Autodesk Inventor part; units mm, degrees
(part 4 of 5)
  arc A546 (145.9727, 136.2043) -> (145.8783, 135.638) centre (153.3985, 134.6758) ccw projected
  arc A547 (146.1603, 136.9638) -> (145.9727, 136.2043) centre (155.6764, 134.2093) ccw projected
  arc A548 (146.4869, 137.9385) -> (146.1603, 136.9638) centre (158.0193, 133.5328) ccw projected
  arc A549 (147.2749, 137.9773) -> (146.4869, 137.9385) centre (148.5, 105) ccw projected
  arc A550 (147.6954, 137.0392) -> (147.2749, 137.9773) centre (136.2299, 132.4624) ccw projected
  arc A551 (147.9566, 136.3017) -> (147.6954, 137.0392) centre (138.4951, 133.3653) ccw projected
  point P0 (0, 0)
fillet "フィレット1" radius 0.5 128 edges at (167.7015, 129.018, -2.5) (168.3105, 128.5182, -2.5) (169.9632, 127.0203, -2.5) (170.5203, 126.4632, -2.5) (165.91, 130.3467, -2.5) (165.2548, 130.7845, -2.5) (163.3417, 131.9311, -2.5) (162.6468, 132.3026, -2.5) (160.6305, 133.2562, -2.5) (159.9026, 133.5577, -2.5) (157.8025, 134.3091, -2.5) (157.0485, 134.5379, -2.5) (154.8849, 135.0798, -2.5) (154.1121, 135.2335, -2.5) (151.9058, 135.5608, -2.5) (151.1217, 135.638, -2.5) (148.894, 135.7475, -2.5) (148.106, 135.7475, -2.5) (145.8783, 135.638, -2.5) (145.0942, 135.5608, -2.5) (142.8879, 135.2335, -2.5) (142.1151, 135.0798, -2.5) (139.9515, 134.5379, -2.5) (139.1975, 134.3091, -2.5) (137.0974, 133.5577, -2.5) (136.3695, 133.2562, -2.5) (134.3532, 132.3026, -2.5) (133.6583, 131.9311, -2.5) (131.7452, 130.7845, -2.5) (131.09, 130.3467, -2.5) (129.2985, 129.018, -2.5) (128.6895, 128.5182, -2.5) (127.0368, 127.0203, -2.5) (126.4797, 126.4632, -2.5) (124.9818, 124.8105, -2.5) (124.482, 124.2015, -2.5) (123.1533, 122.41, -2.5) (122.7155, 121.7548, -2.5) (121.5689, 119.8417, -2.5) (121.1974, 119.1468, -2.5) (120.2438, 117.1305, -2.5) (119.9423, 116.4026, -2.5) (118.9621, 113.5485, -2.5) (119.1909, 114.3025, -2.5) (118.4202, 111.3849, -2.5) (118.2665, 110.6121, -2.5) (117.9392, 108.4058, -2.5) (117.862, 107.6217, -2.5) (117.7525, 105.394, -2.5) (117.7525, 104.606, -2.5) (117.862, 102.3783, -2.5) (117.9392, 101.5942, -2.5) (118.2665, 99.3879, -2.5) (118.4202, 98.6151, -2.5) (118.9621, 96.4515, -2.5) (119.1909, 95.6975, -2.5) (119.9423, 93.5974, -2.5) (120.2438, 92.8695, -2.5) (121.1974, 90.8532, -2.5) (121.5689, 90.1583, -2.5) (122.7155, 88.2452, -2.5) (123.1533, 87.59, -2.5) (124.482, 85.7985, -2.5) (124.9818, 85.1895, -2.5) (126.4797, 83.5368, -2.5) (127.0368, 82.9797, -2.5) (128.6895, 81.4818, -2.5) (129.2985, 80.982, -2.5) (131.09, 79.6533, -2.5) (131.7452, 79.2155, -2.5) (133.6583, 78.0689, -2.5) (134.3532, 77.6974, -2.5) (136.3695, 76.7438, -2.5) (137.0974, 76.4423, -2.5) (139.1975, 75.6909, -2.5) (139.9515, 75.4621, -2.5) (142.1151, 74.9202, -2.5) (142.8879, 74.7665, -2.5) (145.0942, 74.4392, -2.5) (145.8783, 74.362, -2.5) (148.106, 74.2525, -2.5) (151.1217, 74.362, -2.5) (151.9058, 74.4392, -2.5) (148.894, 74.2525, -2.5) (154.1121, 74.7665, -2.5) (154.8849, 74.9202, -2.5) (157.0485, 75.4621, -2.5) (157.8025, 75.6909, -2.5) (159.9026, 76.4423, -2.5) (160.6305, 76.7438, -2.5) (163.3417, 78.0689, -2.5) (162.6468, 77.6974, -2.5) (165.2548, 79.2155, -2.5) (165.91, 79.6533, -2.5) (167.7015, 80.982, -2.5) (168.3105, 81.4818, -2.5) (169.9632, 82.9797, -2.5) (170.5203, 83.5368, -2.5) (172.0182, 85.1895, -2.5) (172.518, 85.7985, -2.5) (173.8467, 87.59, -2.5) (174.2845, 88.2452, -2.5) (175.4311, 90.1583, -2.5) (175.8026, 90.8532, -2.5) (176.7562, 92.8695, -2.5) (177.0577, 93.5974, -2.5) (177.8091, 95.6975, -2.5) (178.0379, 96.4515, -2.5) (178.5798, 98.6151, -2.5) (178.7335, 99.3879, -2.5) (179.0608, 101.5942, -2.5) (179.138, 102.3783, -2.5) (179.2475, 104.606, -2.5) (179.2475, 105.394, -2.5) (179.138, 107.6217, -2.5) (179.0608, 108.4058, -2.5) (178.7335, 110.6121, -2.5) (178.5798, 111.3849, -2.5) (177.8091, 114.3025, -2.5) (178.0379, 113.5485, -2.5) (177.0577, 116.4026, -2.5) (176.7562, 117.1305, -2.5) (175.8026, 119.1468, -2.5) (175.4311, 119.8417, -2.5) (174.2845, 121.7548, -2.5) (173.8467, 122.41, -2.5) (172.518, 124.2015, -2.5) (172.0182, 124.8105, -2.5)
sketch "スケッチ5" plane through (0, 0, 0) normal (0, 0, 1) x (1, 0, 0)
  arc A0 (167.8615, 129.3609) -> (168.0026, 128.7742) centre (168.3197, 129.1607) ccw projected
  arc A1 (168.0126, 128.766) -> (168.0026, 128.7742) centre (148.5, 105) ccw projected
  arc A2 (168.0126, 128.766) -> (168.6156, 128.7421) centre (168.3299, 129.1524) ccw projected
  arc A3 (168.7777, 128.8519) -> (168.6156, 128.7421) centre (172.9477, 122.5201) ccw projected
  arc A4 (169.4474, 129.2562) -> (168.7777, 128.8519) centre (174.2286, 120.5796) ccw projected
  arc A5 (170.3676, 129.7145) -> (169.4474, 129.2562) centre (175.4069, 118.4446) ccw projected
  arc A6 (170.9521, 129.1847) -> (170.3676, 129.7145) centre (148.5, 105) ccw projected
  arc A7 (170.5862, 128.2241) -> (170.9521, 129.1847) centre (159.2425, 133.0951) ccw projected
  arc A8 (170.2495, 127.5179) -> (170.5862, 128.2241) centre (161.4827, 132.1318) ccw projected
  arc A9 (170.1561, 127.3458) -> (170.2495, 127.5179) centre (163.5395, 131.0473) ccw projected
  arc A10 (170.1561, 127.3458) -> (170.239, 126.7481) centre (170.5924, 127.1017) ccw projected
  arc A11 (170.2481, 126.739) -> (170.239, 126.7481) centre (148.5, 105) ccw projected
  arc A12 (170.2481, 126.739) -> (170.8458, 126.6561) centre (170.6017, 127.0924) ccw projected
  arc A13 (171.0179, 126.7495) -> (170.8458, 126.6561) centre (174.5473, 120.0395) ccw projected
  arc A14 (171.7241, 127.0862) -> (171.0179, 126.7495) centre (175.6318, 117.9827) ccw projected
  arc A15 (172.6847, 127.4521) -> (171.7241, 127.0862) centre (176.5951, 115.7425) ccw projected
  arc A16 (173.2145, 126.8676) -> (172.6847, 127.4521) centre (148.5, 105) ccw projected
  arc A17 (172.7562, 125.9474) -> (173.2145, 126.8676) centre (161.9446, 131.9069) ccw projected
  arc A18 (172.3519, 125.2777) -> (172.7562, 125.9474) centre (164.0796, 130.7286) ccw projected
  arc A19 (172.2421, 125.1156) -> (172.3519, 125.2777) centre (166.0201, 129.4477) ccw projected
  arc A20 (172.2421, 125.1156) -> (172.266, 124.5126) centre (172.6524, 124.8299) ccw projected
  arc A21 (172.2742, 124.5026) -> (172.266, 124.5126) centre (148.5, 105) ccw projected
  arc A22 (172.2742, 124.5026) -> (172.8609, 124.3615) centre (172.6607, 124.8197) ccw projected
  arc A23 (173.0413, 124.4376) -> (172.8609, 124.3615) centre (175.896, 117.414) ccw projected
  arc A24 (173.7771, 124.7035) -> (173.0413, 124.4376) centre (176.7737, 115.2608) ccw projected
  arc A25 (174.769, 124.9735) -> (173.7771, 124.7035) centre (177.5128, 112.937) ccw projected
  arc A26 (175.2389, 124.3398) -> (174.769, 124.9735) centre (148.5, 105) ccw projected
  arc A27 (174.6926, 123.469) -> (175.2389, 124.3398) centre (164.5172, 130.4595) ccw projected
  arc A28 (174.2246, 122.8421) -> (174.6926, 123.469) centre (166.5264, 129.0776) ccw projected
  arc A29 (174.0994, 122.6916) -> (174.2246, 122.8421) centre (168.3321, 127.6127) ccw projected
  arc A30 (174.0994, 122.6916) -> (174.0641, 122.0891) centre (174.4798, 122.367) ccw projected
  arc A31 (174.0713, 122.0784) -> (174.0641, 122.0891) centre (148.5, 105) ccw projected
  arc A32 (174.0713, 122.0784) -> (174.6414, 121.8805) centre (174.4871, 122.3561) ccw projected
  arc A33 (174.8283, 121.9385) -> (174.6414, 121.8805) centre (176.9809, 114.6689) ccw projected
  arc A34 (175.5866, 122.131) -> (174.8283, 121.9385) centre (177.6433, 112.4401) ccw projected
  arc A35 (176.6002, 122.3025) -> (175.5866, 122.131) centre (178.151, 110.055) ccw projected
  arc A36 (177.0058, 121.6258) -> (176.6002, 122.3025) centre (148.5, 105) ccw projected
  arc A37 (176.3768, 120.8128) -> (177.0058, 121.6258) centre (166.9355, 128.767) ccw projected
  arc A38 (175.8495, 120.2348) -> (176.3768, 120.8128) centre (168.7996, 127.1948) ccw projected
  arc A39 (175.7102, 120.0972) -> (175.8495, 120.2348) centre (170.453, 125.56) ccw projected
  arc A40 (175.7102, 120.0972) -> (175.616, 119.5011) centre (176.0569, 119.7369) ccw projected
  arc A41 (175.6221, 119.4898) -> (175.616, 119.5011) centre (148.5, 105) ccw projected
  arc A42 (175.6221, 119.4898) -> (176.1701, 119.2369) centre (176.0631, 119.7254) ccw projected
  arc A43 (176.3618, 119.2763) -> (176.1701, 119.2369) centre (177.7914, 111.8308) ccw projected
  arc A44 (177.1353, 119.3936) -> (176.3618, 119.2763) centre (178.2322, 109.5478) ccw projected
  arc A45 (178.1609, 119.4649) -> (177.1353, 119.3936) centre (178.5037, 107.1244) ccw projected
  arc A46 (178.4982, 118.7517) -> (178.1609, 119.4649) centre (148.5, 105) ccw projected
  arc A47 (177.7924, 118.0042) -> (178.4982, 118.7517) centre (169.1763, 126.8455) ccw projected
  arc A48 (177.2111, 117.4807) -> (177.7924, 118.0042) centre (170.8774, 125.0982) ccw projected
  arc A49 (177.059, 117.3574) -> (177.2111, 117.4807) centre (172.3625, 123.3092) ccw projected
  arc A50 (177.059, 117.3574) -> (176.9068, 116.7735) centre (177.3687, 116.9649) ccw projected
  arc A51 (176.9118, 116.7616) -> (176.9068, 116.7735) centre (148.5, 105) ccw projected
  arc A52 (176.9118, 116.7616) -> (177.4323, 116.4562) centre (177.3737, 116.9528) ccw projected
  arc A53 (177.627, 116.4766) -> (177.4323, 116.4562) centre (178.3199, 108.9268) ccw projected
  arc A54 (178.4083, 116.5175) -> (177.627, 116.4766) centre (178.5348, 106.6116) ccw projected
  arc A55 (179.4358, 116.488) -> (178.4083, 116.5175) centre (178.5675, 104.1733) ccw projected
  arc A56 (179.7016, 115.7452) -> (179.4358, 116.488) centre (148.5, 105) ccw projected
  arc A57 (178.926, 115.0704) -> (179.7016, 115.7452) centre (171.218, 124.7137) ccw projected
  arc A58 (178.2962, 114.6064) -> (178.926, 115.0704) centre (172.7396, 122.8081) ccw projected
  arc A59 (178.1327, 114.4987) -> (178.2962, 114.6064) centre (174.0422, 120.8821) ccw projected
  arc A60 (178.1327, 114.4987) -> (177.924, 113.9324) centre (178.4025, 114.0777) ccw projected
  arc A61 (177.9278, 113.9201) -> (177.924, 113.9324) centre (148.5, 105) ccw projected
  arc A62 (177.9278, 113.9201) -> (178.4159, 113.5652) centre (178.4063, 114.0651) ccw projected
  arc A63 (178.6116, 113.5664) -> (178.4159, 113.5652) centre (178.5612, 105.985) ccw projected
  arc A64 (179.3932, 113.5305) -> (178.6116, 113.5664) centre (178.5481, 103.6599) ccw projected
  arc A65 (180.4129, 113.4004) -> (179.3932, 113.5305) centre (178.3417, 101.2301) ccw projected
  arc A66 (180.6046, 112.6351) -> (180.4129, 113.4004) centre (148.5, 105) ccw projected
  arc A67 (179.7666, 112.0397) -> (180.6046, 112.6351) centre (173.0409, 122.392) ccw projected
  arc A68 (179.0943, 111.6396) -> (179.7666, 112.0397) centre (174.3684, 120.3464) ccw projected
  arc A69 (178.9211, 111.5484) -> (179.0943, 111.6396) centre (175.476, 118.302) ccw projected
  arc A70 (178.9211, 111.5484) -> (178.6579, 111.0054) centre (179.1483, 111.103) ccw projected
  arc A71 (178.6604, 110.9927) -> (178.6579, 111.0054) centre (148.5, 105) ccw projected
  arc A72 (178.6604, 110.9927) -> (179.1114, 110.5917) centre (179.1508, 111.0901) ccw projected
  arc A73 (179.3063, 110.5737) -> (179.1114, 110.5917) centre (178.513, 103.0338) ccw projected
  arc A74 (180.0805, 110.4614) -> (179.3063, 110.5737) centre (178.2721, 100.7211) ccw projected
  arc A75 (181.0826, 110.2319) -> (180.0805, 110.4614) centre (177.8285, 98.3233) ccw projected
  arc A76 (181.1984, 109.4516) -> (181.0826, 110.2319) centre (148.5, 105) ccw projected
  arc A77 (180.3061, 108.9411) -> (181.1984, 109.4516) centre (174.6274, 119.9028) ccw projected
  arc A78 (179.5978, 108.6089) -> (180.3061, 108.9411) centre (175.748, 117.737) ccw projected
  arc A79 (179.4164, 108.5351) -> (179.5978, 108.6089) centre (176.6499, 115.5939) ccw projected
  arc A80 (179.4164, 108.5351) -> (179.1013, 108.0204) centre (179.5989, 108.0696) ccw projected
  arc A81 (179.1026, 108.0076) -> (179.1013, 108.0204) centre (148.5, 105) ccw projected
  arc A82 (179.1026, 108.0076) -> (179.512, 107.5643) centre (179.6002, 108.0565) ccw projected
  arc A83 (179.7043, 107.5273) -> (179.512, 107.5643) centre (178.1758, 100.1015) ccw projected
  arc A84 (180.4638, 107.3397) -> (179.7043, 107.5273) centre (177.7093, 97.8236) ccw projected
  arc A85 (181.4385, 107.0131) -> (180.4638, 107.3397) centre (177.0328, 95.4807) ccw projected
  arc A86 (181.4773, 106.2251) -> (181.4385, 107.0131) centre (148.5, 105) ccw projected
  arc A87 (180.5392, 105.8046) -> (181.4773, 106.2251) centre (175.9624, 117.2701) ccw projected
  arc A88 (179.8017, 105.5434) -> (180.5392, 105.8046) centre (176.8653, 115.0049) ccw projected
  arc A89 (179.6141, 105.4877) -> (179.8017, 105.5434) centre (177.5527, 112.7837) ccw projected
  arc A90 (179.6141, 105.4877) -> (179.25, 105.0065) centre (179.75, 105.0066) ccw projected
  arc A91 (179.25, 104.9935) -> (179.25, 105.0065) centre (148.5, 105) ccw projected
  arc A92 (179.25, 104.9935) -> (179.6141, 104.5123) centre (179.75, 104.9934) ccw projected
  arc A93 (179.8017, 104.4566) -> (179.6141, 104.5123) centre (177.5527, 97.2163) ccw projected
  arc A94 (180.5392, 104.1954) -> (179.8017, 104.4566) centre (176.8653, 94.9951) ccw projected
  arc A95 (181.4773, 103.7749) -> (180.5392, 104.1954) centre (175.9624, 92.7299) ccw projected
  arc A96 (181.4385, 102.9869) -> (181.4773, 103.7749) centre (148.5, 105) ccw projected
  arc A97 (180.4638, 102.6603) -> (181.4385, 102.9869) centre (177.0328, 114.5193) ccw projected
  arc A98 (179.7043, 102.4727) -> (180.4638, 102.6603) centre (177.7093, 112.1764) ccw projected
  arc A99 (179.512, 102.4357) -> (179.7043, 102.4727) centre (178.1758, 109.8985) ccw projected
  arc A100 (179.512, 102.4357) -> (179.1026, 101.9924) centre (179.6002, 101.9435) ccw projected
  arc A101 (179.1013, 101.9796) -> (179.1026, 101.9924) centre (148.5, 105) ccw projected
  arc A102 (179.1013, 101.9796) -> (179.4164, 101.4649) centre (179.5989, 101.9304) ccw projected
  arc A103 (179.5978, 101.3911) -> (179.4164, 101.4649) centre (176.6499, 94.4061) ccw projected
  arc A104 (180.3061, 101.0589) -> (179.5978, 101.3911) centre (175.748, 92.263) ccw projected
  arc A105 (181.1984, 100.5484) -> (180.3061, 101.0589) centre (174.6274, 90.0972) ccw projected
  arc A106 (181.0826, 99.7681) -> (181.1984, 100.5484) centre (148.5, 105) ccw projected
  arc A107 (180.0805, 99.5386) -> (181.0826, 99.7681) centre (177.8285, 111.6767) ccw projected
  arc A108 (179.3063, 99.4263) -> (180.0805, 99.5386) centre (178.2721, 109.2789) ccw projected
  arc A109 (179.1114, 99.4083) -> (179.3063, 99.4263) centre (178.513, 106.9662) ccw projected
  arc A110 (179.1114, 99.4083) -> (178.6604, 99.0073) centre (179.1508, 98.9099) ccw projected
  arc A111 (178.6579, 98.9946) -> (178.6604, 99.0073) centre (148.5, 105) ccw projected
  arc A112 (178.6579, 98.9946) -> (178.9211, 98.4516) centre (179.1483, 98.897) ccw projected
  arc A113 (179.0943, 98.3604) -> (178.9211, 98.4516) centre (175.476, 91.698) ccw projected
  arc A114 (179.7666, 97.9603) -> (179.0943, 98.3604) centre (174.3684, 89.6536) ccw projected
  arc A115 (180.6046, 97.3649) -> (179.7666, 97.9603) centre (173.0409, 87.608) ccw projected
  arc A116 (180.4129, 96.5996) -> (180.6046, 97.3649) centre (148.5, 105) ccw projected
  arc A117 (179.3932, 96.4695) -> (180.4129, 96.5996) centre (178.3417, 108.7699) ccw projected
  arc A118 (178.6116, 96.4336) -> (179.3932, 96.4695) centre (178.5481, 106.3401) ccw projected
  arc A119 (178.4159, 96.4348) -> (178.6116, 96.4336) centre (178.5612, 104.015) ccw projected
  arc A120 (178.4159, 96.4348) -> (177.9278, 96.0799) centre (178.4063, 95.9349) ccw projected
  arc A121 (177.924, 96.0676) -> (177.9278, 96.0799) centre (148.5, 105) ccw projected
  arc A122 (177.924, 96.0676) -> (178.1327, 95.5013) centre (178.4025, 95.9223) ccw projected
  arc A123 (178.2962, 95.3936) -> (178.1327, 95.5013) centre (174.0422, 89.1179) ccw projected
  arc A124 (178.926, 94.9296) -> (178.2962, 95.3936) centre (172.7396, 87.1919) ccw projected
  arc A125 (179.7016, 94.2548) -> (178.926, 94.9296) centre (171.218, 85.2863) ccw projected
  arc A126 (179.4358, 93.512) -> (179.7016, 94.2548) centre (148.5, 105) ccw projected
  arc A127 (178.4083, 93.4825) -> (179.4358, 93.512) centre (178.5675, 105.8267) ccw projected
  arc A128 (177.627, 93.5234) -> (178.4083, 93.4825) centre (178.5348, 103.3884) ccw projected
  arc A129 (177.4323, 93.5438) -> (177.627, 93.5234) centre (178.3199, 101.0732) ccw projected
  arc A130 (177.4323, 93.5438) -> (176.9118, 93.2384) centre (177.3737, 93.0472) ccw projected
  arc A131 (176.9068, 93.2265) -> (176.9118, 93.2384) centre (148.5, 105) ccw projected
  arc A132 (176.9068, 93.2265) -> (177.059, 92.6426) centre (177.3687, 93.0351) ccw projected
  arc A133 (177.2111, 92.5193) -> (177.059, 92.6426) centre (172.3625, 86.6908) ccw projected
  arc A134 (177.7924, 91.9958) -> (177.2111, 92.5193) centre (170.8774, 84.9018) ccw projected
  arc A135 (178.4982, 91.2483) -> (177.7924, 91.9958) centre (169.1763, 83.1545) ccw projected
  arc A136 (178.1609, 90.5351) -> (178.4982, 91.2483) centre (148.5, 105) ccw projected
  arc A137 (177.1353, 90.6064) -> (178.1609, 90.5351) centre (178.5037, 102.8756) ccw projected
  arc A138 (176.3618, 90.7237) -> (177.1353, 90.6064) centre (178.2322, 100.4522) ccw projected
  arc A139 (176.1701, 90.7631) -> (176.3618, 90.7237) centre (177.7914, 98.1692) ccw projected
  arc A140 (176.1701, 90.7631) -> (175.6221, 90.5102) centre (176.0631, 90.2746) ccw projected
  arc A141 (175.616, 90.4989) -> (175.6221, 90.5102) centre (148.5, 105) ccw projected
  arc A142 (175.616, 90.4989) -> (175.7102, 89.9028) centre (176.0569, 90.2631) ccw projected
  arc A143 (175.8495, 89.7652) -> (175.7102, 89.9028) centre (170.453, 84.44) ccw projected
  arc A144 (176.3768, 89.1872) -> (175.8495, 89.7652) centre (168.7996, 82.8052) ccw projected
  arc A145 (177.0058, 88.3742) -> (176.3768, 89.1872) centre (166.9355, 81.233) ccw projected
  arc A146 (176.6002, 87.6975) -> (177.0058, 88.3742) centre (148.5, 105) ccw projected
  arc A147 (175.5866, 87.869) -> (176.6002, 87.6975) centre (178.151, 99.945) ccw projected
  arc A148 (174.8283, 88.0615) -> (175.5866, 87.869) centre (177.6433, 97.5599) ccw projected
  arc A149 (174.6414, 88.1195) -> (174.8283, 88.0615) centre (176.9809, 95.3311) ccw projected
  arc A150 (174.6414, 88.1195) -> (174.0713, 87.9216) centre (174.4871, 87.6439) ccw projected
  arc A151 (174.0641, 87.9109) -> (174.0713, 87.9216) centre (148.5, 105) ccw projected
  arc A152 (174.0641, 87.9109) -> (174.0994, 87.3084) centre (174.4798, 87.633) ccw projected
  arc A153 (174.2246, 87.1579) -> (174.0994, 87.3084) centre (168.3321, 82.3873) ccw projected
  arc A154 (174.6926, 86.531) -> (174.2246, 87.1579) centre (166.5264, 80.9224) ccw projected
  arc A155 (175.2389, 85.6602) -> (174.6926, 86.531) centre (164.5172, 79.5405) ccw projected
  arc A156 (174.769, 85.0265) -> (175.2389, 85.6602) centre (148.5, 105) ccw projected
  arc A157 (173.7771, 85.2965) -> (174.769, 85.0265) centre (177.5128, 97.063) ccw projected
  arc A158 (173.0413, 85.5624) -> (173.7771, 85.2965) centre (176.7737, 94.7392) ccw projected
  arc A159 (172.8609, 85.6385) -> (173.0413, 85.5624) centre (175.896, 92.586) ccw projected
  arc A160 (172.8609, 85.6385) -> (172.2742, 85.4974) centre (172.6607, 85.1803) ccw projected
  arc A161 (172.266, 85.4874) -> (172.2742, 85.4974) centre (148.5, 105) ccw projected
  arc A162 (172.266, 85.4874) -> (172.2421, 84.8844) centre (172.6524, 85.1701) ccw projected
  arc A163 (172.3519, 84.7223) -> (172.2421, 84.8844) centre (166.0201, 80.5523) ccw projected
  arc A164 (172.7562, 84.0526) -> (172.3519, 84.7223) centre (164.0796, 79.2714) ccw projected
  arc A165 (173.2145, 83.1324) -> (172.7562, 84.0526) centre (161.9446, 78.0931) ccw projected
  arc A166 (172.6847, 82.5479) -> (173.2145, 83.1324) centre (148.5, 105) ccw projected
  arc A167 (171.7241, 82.9138) -> (172.6847, 82.5479) centre (176.5951, 94.2575) ccw projected
  arc A168 (171.0179, 83.2505) -> (171.7241, 82.9138) centre (175.6318, 92.0173) ccw projected
  arc A169 (170.8458, 83.3439) -> (171.0179, 83.2505) centre (174.5473, 89.9605) ccw projected
  arc A170 (170.8458, 83.3439) -> (170.2481, 83.261) centre (170.6017, 82.9076) ccw projected
  arc A171 (170.239, 83.2519) -> (170.2481, 83.261) centre (148.5, 105) ccw projected
  arc A172 (170.239, 83.2519) -> (170.1561, 82.6542) centre (170.5924, 82.8983) ccw projected
  arc A173 (170.2495, 82.4821) -> (170.1561, 82.6542) centre (163.5395, 78.9527) ccw projected
  arc A174 (170.5862, 81.7759) -> (170.2495, 82.4821) centre (161.4827, 77.8682) ccw projected
  arc A175 (170.9521, 80.8153) -> (170.5862, 81.7759) centre (159.2425, 76.9049) ccw projected
  arc A176 (170.3676, 80.2855) -> (170.9521, 80.8153) centre (148.5, 105) ccw projected
  arc A177 (169.4474, 80.7438) -> (170.3676, 80.2855) centre (175.4069, 91.5554) ccw projected
  arc A178 (168.7777, 81.1481) -> (169.4474, 80.7438) centre (174.2286, 89.4204) ccw projected
  arc A179 (168.6156, 81.2579) -> (168.7777, 81.1481) centre (172.9477, 87.4799) ccw projected
  arc A180 (168.6156, 81.2579) -> (168.0126, 81.234) centre (168.3299, 80.8476) ccw projected
  arc A181 (168.0026, 81.2258) -> (168.0126, 81.234) centre (148.5, 105) ccw projected
  arc A182 (168.0026, 81.2258) -> (167.8615, 80.6391) centre (168.3197, 80.8393) ccw projected
  arc A183 (167.9376, 80.4587) -> (167.8615, 80.6391) centre (160.914, 77.604) ccw projected
  arc A184 (168.2035, 79.7229) -> (167.9376, 80.4587) centre (158.7608, 76.7263) ccw projected
  arc A185 (168.4735, 78.731) -> (168.2035, 79.7229) centre (156.437, 75.9872) ccw projected
  arc A186 (167.8398, 78.2611) -> (168.4735, 78.731) centre (148.5, 105) ccw projected
  arc A187 (166.969, 78.8074) -> (167.8398, 78.2611) centre (173.9595, 88.9828) ccw projected
  arc A188 (166.3421, 79.2754) -> (166.969, 78.8074) centre (172.5776, 86.9736) ccw projected
  arc A189 (166.1916, 79.4006) -> (166.3421, 79.2754) centre (171.1127, 85.1679) ccw projected
  arc A190 (166.1916, 79.4006) -> (165.5891, 79.4359) centre (165.867, 79.0202) ccw projected
  arc A191 (165.5784, 79.4287) -> (165.5891, 79.4359) centre (148.5, 105) ccw projected
  arc A192 (165.5784, 79.4287) -> (165.3805, 78.8586) centre (165.8561, 79.0129) ccw projected
  arc A193 (165.4385, 78.6717) -> (165.3805, 78.8586) centre (158.1689, 76.5191) ccw projected
  arc A194 (165.631, 77.9134) -> (165.4385, 78.6717) centre (155.9401, 75.8567) ccw projected
  arc A195 (165.8025, 76.8998) -> (165.631, 77.9134) centre (153.555, 75.349) ccw projected
  arc A196 (165.1258, 76.4942) -> (165.8025, 76.8998) centre (148.5, 105) ccw projected
  arc A197 (164.3128, 77.1232) -> (165.1258, 76.4942) centre (172.267, 86.5645) ccw projected
  arc A198 (163.7348, 77.6505) -> (164.3128, 77.1232) centre (170.6948, 84.7004) ccw projected
  arc A199 (163.5972, 77.7898) -> (163.7348, 77.6505) centre (169.06, 83.047) ccw projected
  arc A200 (163.5972, 77.7898) -> (163.0011, 77.884) centre (163.2369, 77.4431) ccw projected
  arc A201 (162.9898, 77.8779) -> (163.0011, 77.884) centre (148.5, 105) ccw projected
  arc A202 (162.9898, 77.8779) -> (162.7369, 77.3299) centre (163.2254, 77.4369) ccw projected
  arc A203 (162.7763, 77.1382) -> (162.7369, 77.3299) centre (155.3308, 75.7086) ccw projected
  arc A204 (162.8936, 76.3647) -> (162.7763, 77.1382) centre (153.0478, 75.2678) ccw projected
  arc A205 (162.9649, 75.3391) -> (162.8936, 76.3647) centre (150.6244, 74.9963) ccw projected
  arc A206 (162.2517, 75.0018) -> (162.9649, 75.3391) centre (148.5, 105) ccw projected
  arc A207 (161.5042, 75.7076) -> (162.2517, 75.0018) centre (170.3455, 84.3237) ccw projected
  arc A208 (160.9807, 76.2889) -> (161.5042, 75.7076) centre (168.5982, 82.6226) ccw projected
  arc A209 (160.8574, 76.441) -> (160.9807, 76.2889) centre (166.8092, 81.1375) ccw projected
  arc A210 (160.8574, 76.441) -> (160.2735, 76.5932) centre (160.4649, 76.1313) ccw projected
  arc A211 (160.2616, 76.5882) -> (160.2735, 76.5932) centre (148.5, 105) ccw projected
  arc A212 (160.2616, 76.5882) -> (159.9562, 76.0677) centre (160.4528, 76.1263) ccw projected
  arc A213 (159.9766, 75.873) -> (159.9562, 76.0677) centre (152.4268, 75.1801) ccw projected
  arc A214 (160.0175, 75.0917) -> (159.9766, 75.873) centre (150.1116, 74.9652) ccw projected
  arc A215 (159.988, 74.0642) -> (160.0175, 75.0917) centre (147.6733, 74.9325) ccw projected
  arc A216 (159.2452, 73.7984) -> (159.988, 74.0642) centre (148.5, 105) ccw projected
  arc A217 (158.5704, 74.574) -> (159.2452, 73.7984) centre (168.2137, 82.282) ccw projected
  arc A218 (158.1064, 75.2038) -> (158.5704, 74.574) centre (166.3081, 80.7604) ccw projected
  arc A219 (157.9987, 75.3673) -> (158.1064, 75.2038) centre (164.3821, 79.4578) ccw projected
  arc A220 (157.9987, 75.3673) -> (157.4324, 75.576) centre (157.5777, 75.0975) ccw projected
  arc A221 (157.4201, 75.5722) -> (157.4324, 75.576) centre (148.5, 105) ccw projected
  arc A222 (157.4201, 75.5722) -> (157.0652, 75.0841) centre (157.5651, 75.0937) ccw projected
  arc A223 (157.0664, 74.8884) -> (157.0652, 75.0841) centre (149.485, 74.9388) ccw projected
  arc A224 (157.0305, 74.1068) -> (157.0664, 74.8884) centre (147.1599, 74.9519) ccw projected
  arc A225 (156.9004, 73.0871) -> (157.0305, 74.1068) centre (144.7301, 75.1583) ccw projected
  arc A226 (156.1351, 72.8954) -> (156.9004, 73.0871) centre (148.5, 105) ccw projected
  arc A227 (155.5397, 73.7334) -> (156.1351, 72.8954) centre (165.892, 80.4591) ccw projected
  arc A228 (155.1396, 74.4057) -> (155.5397, 73.7334) centre (163.8464, 79.1316) ccw projected
  arc A229 (155.0484, 74.5789) -> (155.1396, 74.4057) centre (161.802, 78.024) ccw projected
  arc A230 (155.0484, 74.5789) -> (154.5054, 74.8421) centre (154.603, 74.3517) ccw projected
  arc A231 (154.4927, 74.8396) -> (154.5054, 74.8421) centre (148.5, 105) ccw projected
  arc A232 (154.4927, 74.8396) -> (154.0917, 74.3886) centre (154.5901, 74.3492) ccw projected
  arc A233 (154.0737, 74.1937) -> (154.0917, 74.3886) centre (146.5338, 74.987) ccw projected
  arc A234 (153.9614, 73.4195) -> (154.0737, 74.1937) centre (144.2211, 75.2279) ccw projected
  arc A235 (153.7319, 72.4174) -> (153.9614, 73.4195) centre (141.8233, 75.6715) ccw projected
  arc A236 (152.9516, 72.3016) -> (153.7319, 72.4174) centre (148.5, 105) ccw projected
  arc A237 (152.4411, 73.1939) -> (152.9516, 72.3016) centre (163.4028, 78.8726) ccw projected
  arc A238 (152.1089, 73.9022) -> (152.4411, 73.1939) centre (161.237, 77.752) ccw projected
  arc A239 (152.0351, 74.0836) -> (152.1089, 73.9022) centre (159.0939, 76.8501) ccw projected
  arc A240 (152.0351, 74.0836) -> (151.5204, 74.3987) centre (151.5696, 73.9011) ccw projected
  arc A241 (151.5076, 74.3974) -> (151.5204, 74.3987) centre (148.5, 105) ccw projected
  arc A242 (151.5076, 74.3974) -> (151.0643, 73.988) centre (151.5565, 73.8998) ccw projected
  arc A243 (151.0273, 73.7957) -> (151.0643, 73.988) centre (143.6015, 75.3242) ccw projected
  arc A244 (150.8397, 73.0362) -> (151.0273, 73.7957) centre (141.3236, 75.7907) ccw projected
  arc A245 (150.5131, 72.0615) -> (150.8397, 73.0362) centre (138.9807, 76.4672) ccw projected
  arc A246 (149.7251, 72.0227) -> (150.5131, 72.0615) centre (148.5, 105) ccw projected
  arc A247 (149.3046, 72.9608) -> (149.7251, 72.0227) centre (160.7701, 77.5376) ccw projected
  arc A248 (149.0434, 73.6983) -> (149.3046, 72.9608) centre (158.5049, 76.6347) ccw projected
  arc A249 (148.9877, 73.8859) -> (149.0434, 73.6983) centre (156.2837, 75.9473) ccw projected
  arc A250 (148.9877, 73.8859) -> (148.5065, 74.25) centre (148.5066, 73.75) ccw projected
  arc A251 (148.4935, 74.25) -> (148.5065, 74.25) centre (148.5, 105) ccw projected
  arc A252 (148.4935, 74.25) -> (148.0123, 73.8859) centre (148.4934, 73.75) ccw projected
  arc A253 (147.9566, 73.6983) -> (148.0123, 73.8859) centre (140.7163, 75.9473) ccw projected
  arc A254 (147.6954, 72.9608) -> (147.9566, 73.6983) centre (138.4951, 76.6347) ccw projected
  arc A255 (147.2749, 72.0227) -> (147.6954, 72.9608) centre (136.2299, 77.5376) ccw projected
  arc A256 (146.4869, 72.0615) -> (147.2749, 72.0227) centre (148.5, 105) ccw projected
  arc A257 (146.1603, 73.0362) -> (146.4869, 72.0615) centre (158.0193, 76.4672) ccw projected
  arc A258 (145.9727, 73.7957) -> (146.1603, 73.0362) centre (155.6764, 75.7907) ccw projected
  arc A259 (145.9357, 73.988) -> (145.9727, 73.7957) centre (153.3985, 75.3242) ccw projected
  arc A260 (145.9357, 73.988) -> (145.4924, 74.3974) centre (145.4435, 73.8998) ccw projected
  arc A261 (145.4796, 74.3987) -> (145.4924, 74.3974) centre (148.5, 105) ccw projected
  arc A262 (145.4796, 74.3987) -> (144.9649, 74.0836) centre (145.4304, 73.9011) ccw projected
  arc A263 (144.8911, 73.9022) -> (144.9649, 74.0836) centre (137.9061, 76.8501) ccw projected
  arc A264 (144.5589, 73.1939) -> (144.8911, 73.9022) centre (135.763, 77.752) ccw projected
  arc A265 (144.0484, 72.3016) -> (144.5589, 73.1939) centre (133.5972, 78.8726) ccw projected
  arc A266 (143.2681, 72.4174) -> (144.0484, 72.3016) centre (148.5, 105) ccw projected
  arc A267 (143.0386, 73.4195) -> (143.2681, 72.4174) centre (155.1767, 75.6715) ccw projected
  arc A268 (142.9263, 74.1937) -> (143.0386, 73.4195) centre (152.7789, 75.2279) ccw projected
  arc A269 (142.9083, 74.3886) -> (142.9263, 74.1937) centre (150.4662, 74.987) ccw projected
  arc A270 (142.9083, 74.3886) -> (142.5073, 74.8396) centre (142.4099, 74.3492) ccw projected
  arc A271 (142.4946, 74.8421) -> (142.5073, 74.8396) centre (148.5, 105) ccw projected
  arc A272 (142.4946, 74.8421) -> (141.9516, 74.5789) centre (142.397, 74.3517) ccw projected
  arc A273 (141.8604, 74.4057) -> (141.9516, 74.5789) centre (135.198, 78.024) ccw projected
  arc A274 (141.4603, 73.7334) -> (141.8604, 74.4057) centre (133.1536, 79.1316) ccw projected
  arc A275 (140.8649, 72.8954) -> (141.4603, 73.7334) centre (131.108, 80.4591) ccw projected
  arc A276 (140.0996, 73.0871) -> (140.8649, 72.8954) centre (148.5, 105) ccw projected
  arc A277 (139.9695, 74.1068) -> (140.0996, 73.0871) centre (152.2699, 75.1583) ccw projected
  arc A278 (139.9336, 74.8884) -> (139.9695, 74.1068) centre (149.8401, 74.9519) ccw projected
  arc A279 (139.9348, 75.0841) -> (139.9336, 74.8884) centre (147.515, 74.9388) ccw projected
  arc A280 (139.9348, 75.0841) -> (139.5799, 75.5722) centre (139.4349, 75.0937) ccw projected
  arc A281 (139.5676, 75.576) -> (139.5799, 75.5722) centre (148.5, 105) ccw projected
  arc A282 (139.5676, 75.576) -> (139.0013, 75.3673) centre (139.4223, 75.0975) ccw projected
  arc A283 (138.8936, 75.2038) -> (139.0013, 75.3673) centre (132.6179, 79.4578) ccw projected
  arc A284 (138.4296, 74.574) -> (138.8936, 75.2038) centre (130.6919, 80.7604) ccw projected
  arc A285 (137.7548, 73.7984) -> (138.4296, 74.574) centre (128.7863, 82.282) ccw projected
  arc A286 (137.012, 74.0642) -> (137.7548, 73.7984) centre (148.5, 105) ccw projected
  arc A287 (136.9825, 75.0917) -> (137.012, 74.0642) centre (149.3267, 74.9325) ccw projected
  arc A288 (137.0234, 75.873) -> (136.9825, 75.0917) centre (146.8884, 74.9652) ccw projected
  arc A289 (137.0438, 76.0677) -> (137.0234, 75.873) centre (144.5732, 75.1801) ccw projected
  arc A290 (137.0438, 76.0677) -> (136.7384, 76.5882) centre (136.5472, 76.1263) ccw projected
  arc A291 (136.7265, 76.5932) -> (136.7384, 76.5882) centre (148.5, 105) ccw projected
  arc A292 (136.7265, 76.5932) -> (136.1426, 76.441) centre (136.5351, 76.1313) ccw projected
  arc A293 (136.0193, 76.2889) -> (136.1426, 76.441) centre (130.1908, 81.1375) ccw projected
  arc A294 (135.4958, 75.7076) -> (136.0193, 76.2889) centre (128.4018, 82.6226) ccw projected
  arc A295 (134.7483, 75.0018) -> (135.4958, 75.7076) centre (126.6545, 84.3237) ccw projected
  arc A296 (134.0351, 75.3391) -> (134.7483, 75.0018) centre (148.5, 105) ccw projected
  arc A297 (134.1064, 76.3647) -> (134.0351, 75.3391) centre (146.3756, 74.9963) ccw projected
  arc A298 (134.2237, 77.1382) -> (134.1064, 76.3647) centre (143.9522, 75.2678) ccw projected
  arc A299 (134.2631, 77.3299) -> (134.2237, 77.1382) centre (141.6692, 75.7086) ccw projected
  arc A300 (134.2631, 77.3299) -> (134.0102, 77.8779) centre (133.7746, 77.4369) ccw projected
  arc A301 (133.9989, 77.884) -> (134.0102, 77.8779) centre (148.5, 105) ccw projected
  arc A302 (133.9989, 77.884) -> (133.4028, 77.7898) centre (133.7631, 77.4431) ccw projected
  arc A303 (133.2652, 77.6505) -> (133.4028, 77.7898) centre (127.94, 83.047) ccw projected
  arc A304 (132.6872, 77.1232) -> (133.2652, 77.6505) centre (126.3052, 84.7004) ccw projected
  arc A305 (131.8742, 76.4942) -> (132.6872, 77.1232) centre (124.733, 86.5645) ccw projected
  arc A306 (131.1975, 76.8998) -> (131.8742, 76.4942) centre (148.5, 105) ccw projected
  arc A307 (131.369, 77.9134) -> (131.1975, 76.8998) centre (143.445, 75.349) ccw projected
  arc A308 (131.5615, 78.6717) -> (131.369, 77.9134) centre (141.0599, 75.8567) ccw projected
  arc A309 (131.6195, 78.8586) -> (131.5615, 78.6717) centre (138.8311, 76.5191) ccw projected
  arc A310 (131.6195, 78.8586) -> (131.4216, 79.4287) centre (131.1439, 79.0129) ccw projected
  arc A311 (131.4109, 79.4359) -> (131.4216, 79.4287) centre (148.5, 105) ccw projected
  arc A312 (131.4109, 79.4359) -> (130.8084, 79.4006) centre (131.133, 79.0202) ccw projected
  arc A313 (130.6579, 79.2754) -> (130.8084, 79.4006) centre (125.8873, 85.1679) ccw projected
  arc A314 (130.031, 78.8074) -> (130.6579, 79.2754) centre (124.4224, 86.9736) ccw projected
  arc A315 (129.1602, 78.2611) -> (130.031, 78.8074) centre (123.0405, 88.9828) ccw projected
  arc A316 (128.5265, 78.731) -> (129.1602, 78.2611) centre (148.5, 105) ccw projected
  arc A317 (128.7965, 79.7229) -> (128.5265, 78.731) centre (140.563, 75.9872) ccw projected
  arc A318 (129.0624, 80.4587) -> (128.7965, 79.7229) centre (138.2392, 76.7263) ccw projected
  arc A319 (129.1385, 80.6391) -> (129.0624, 80.4587) centre (136.086, 77.604) ccw projected
  arc A320 (129.1385, 80.6391) -> (128.9974, 81.2258) centre (128.6803, 80.8393) ccw projected
  arc A321 (128.9874, 81.234) -> (128.9974, 81.2258) centre (148.5, 105) ccw projected
  arc A322 (128.9874, 81.234) -> (128.3844, 81.2579) centre (128.6701, 80.8476) ccw projected
  arc A323 (128.2223, 81.1481) -> (128.3844, 81.2579) centre (124.0523, 87.4799) ccw projected
  arc A324 (127.5526, 80.7438) -> (128.2223, 81.1481) centre (122.7714, 89.4204) ccw projected
  arc A325 (126.6324, 80.2855) -> (127.5526, 80.7438) centre (121.5931, 91.5554) ccw projected
  arc A326 (126.0479, 80.8153) -> (126.6324, 80.2855) centre (148.5, 105) ccw projected
  arc A327 (126.4138, 81.7759) -> (126.0479, 80.8153) centre (137.7575, 76.9049) ccw projected
  arc A328 (126.7505, 82.4821) -> (126.4138, 81.7759) centre (135.5173, 77.8682) ccw projected
  arc A329 (126.8439, 82.6542) -> (126.7505, 82.4821) centre (133.4605, 78.9527) ccw projected
  arc A330 (126.8439, 82.6542) -> (126.761, 83.2519) centre (126.4076, 82.8983) ccw projected
  arc A331 (126.7519, 83.261) -> (126.761, 83.2519) centre (148.5, 105) ccw projected
  arc A332 (126.7519, 83.261) -> (126.1542, 83.3439) centre (126.3983, 82.9076) ccw projected
  arc A333 (125.9821, 83.2505) -> (126.1542, 83.3439) centre (122.4527, 89.9605) ccw projected
  arc A334 (125.2759, 82.9138) -> (125.9821, 83.2505) centre (121.3682, 92.0173) ccw projected
  arc A335 (124.3153, 82.5479) -> (125.2759, 82.9138) centre (120.4049, 94.2575) ccw projected
  arc A336 (123.7855, 83.1324) -> (124.3153, 82.5479) centre (148.5, 105) ccw projected
  arc A337 (124.2438, 84.0526) -> (123.7855, 83.1324) centre (135.0554, 78.0931) ccw projected
  arc A338 (124.6481, 84.7223) -> (124.2438, 84.0526) centre (132.9204, 79.2714) ccw projected
  arc A339 (124.7579, 84.8844) -> (124.6481, 84.7223) centre (130.9799, 80.5523) ccw projected
  arc A340 (124.7579, 84.8844) -> (124.734, 85.4874) centre (124.3476, 85.1701) ccw projected
  arc A341 (124.7258, 85.4974) -> (124.734, 85.4874) centre (148.5, 105) ccw projected
  arc A342 (124.7258, 85.4974) -> (124.1391, 85.6385) centre (124.3393, 85.1803) ccw projected
  arc A343 (123.9587, 85.5624) -> (124.1391, 85.6385) centre (121.104, 92.586) ccw projected
  arc A344 (123.2229, 85.2965) -> (123.9587, 85.5624) centre (120.2263, 94.7392) ccw projected
  arc A345 (122.231, 85.0265) -> (123.2229, 85.2965) centre (119.4872, 97.063) ccw projected
  arc A346 (121.7611, 85.6602) -> (122.231, 85.0265) centre (148.5, 105) ccw projected
  arc A347 (122.3074, 86.531) -> (121.7611, 85.6602) centre (132.4828, 79.5405) ccw projected
  arc A348 (122.7754, 87.1579) -> (122.3074, 86.531) centre (130.4736, 80.9224) ccw projected
  arc A349 (122.9006, 87.3084) -> (122.7754, 87.1579) centre (128.6679, 82.3873) ccw projected
  arc A350 (122.9006, 87.3084) -> (122.9359, 87.9109) centre (122.5202, 87.633) ccw projected
  arc A351 (122.9287, 87.9216) -> (122.9359, 87.9109) centre (148.5, 105) ccw projected
  arc A352 (122.9287, 87.9216) -> (122.3586, 88.1195) centre (122.5129, 87.6439) ccw projected
  arc A353 (122.1717, 88.0615) -> (122.3586, 88.1195) centre (120.0191, 95.3311) ccw projected
  arc A354 (121.4134, 87.869) -> (122.1717, 88.0615) centre (119.3567, 97.5599) ccw projected
  arc A355 (120.3998, 87.6975) -> (121.4134, 87.869) centre (118.849, 99.945) ccw projected
  arc A356 (119.9942, 88.3742) -> (120.3998, 87.6975) centre (148.5, 105) ccw projected
  arc A357 (120.6232, 89.1872) -> (119.9942, 88.3742) centre (130.0645, 81.233) ccw projected
  arc A358 (121.1505, 89.7652) -> (120.6232, 89.1872) centre (128.2004, 82.8052) ccw projected
  arc A359 (121.2898, 89.9028) -> (121.1505, 89.7652) centre (126.547, 84.44) ccw projected
  arc A360 (121.2898, 89.9028) -> (121.384, 90.4989) centre (120.9431, 90.2631) ccw projected
  arc A361 (121.3779, 90.5102) -> (121.384, 90.4989) centre (148.5, 105) ccw projected
  arc A362 (121.3779, 90.5102) -> (120.8299, 90.7631) centre (120.9369, 90.2746) ccw projected
  arc A363 (120.6382, 90.7237) -> (120.8299, 90.7631) centre (119.2086, 98.1692) ccw projected
  arc A364 (119.8647, 90.6064) -> (120.6382, 90.7237) centre (118.7678, 100.4522) ccw projected
  arc A365 (118.8391, 90.5351) -> (119.8647, 90.6064) centre (118.4963, 102.8756) ccw projected
  arc A366 (118.5018, 91.2483) -> (118.8391, 90.5351) centre (148.5, 105) ccw projected
  arc A367 (119.2076, 91.9958) -> (118.5018, 91.2483) centre (127.8237, 83.1545) ccw projected
  arc A368 (119.7889, 92.5193) -> (119.2076, 91.9958) centre (126.1226, 84.9018) ccw projected
  arc A369 (119.941, 92.6426) -> (119.7889, 92.5193) centre (124.6375, 86.6908) ccw projected
  arc A370 (119.941, 92.6426) -> (120.0932, 93.2265) centre (119.6313, 93.0351) ccw projected
  arc A371 (120.0882, 93.2384) -> (120.0932, 93.2265) centre (148.5, 105) ccw projected
  arc A372 (120.0882, 93.2384) -> (119.5677, 93.5438) centre (119.6263, 93.0472) ccw projected
  arc A373 (119.373, 93.5234) -> (119.5677, 93.5438) centre (118.6801, 101.0732) ccw projected
  arc A374 (118.5917, 93.4825) -> (119.373, 93.5234) centre (118.4652, 103.3884) ccw projected
  arc A375 (117.5642, 93.512) -> (118.5917, 93.4825) centre (118.4325, 105.8267) ccw projected
  arc A376 (117.2984, 94.2548) -> (117.5642, 93.512) centre (148.5, 105) ccw projected
  arc A377 (118.074, 94.9296) -> (117.2984, 94.2548) centre (125.782, 85.2863) ccw projected
  arc A378 (118.7038, 95.3936) -> (118.074, 94.9296) centre (124.2604, 87.1919) ccw projected
  arc A379 (118.8673, 95.5013) -> (118.7038, 95.3936) centre (122.9578, 89.1179) ccw projected
  arc A380 (118.8673, 95.5013) -> (119.076, 96.0676) centre (118.5975, 95.9223) ccw projected
  arc A381 (119.0722, 96.0799) -> (119.076, 96.0676) centre (148.5, 105) ccw projected
  arc A382 (119.0722, 96.0799) -> (118.5841, 96.4348) centre (118.5937, 95.9349) ccw projected
  arc A383 (118.3884, 96.4336) -> (118.5841, 96.4348) centre (118.4388, 104.015) ccw projected
  arc A384 (117.6068, 96.4695) -> (118.3884, 96.4336) centre (118.4519, 106.3401) ccw projected
  arc A385 (116.5871, 96.5996) -> (117.6068, 96.4695) centre (118.6583, 108.7699) ccw projected
  arc A386 (116.3954, 97.3649) -> (116.5871, 96.5996) centre (148.5, 105) ccw projected
  arc A387 (117.2334, 97.9603) -> (116.3954, 97.3649) centre (123.9591, 87.608) ccw projected
  arc A388 (117.9057, 98.3604) -> (117.2334, 97.9603) centre (122.6316, 89.6536) ccw projected
  arc A389 (118.0789, 98.4516) -> (117.9057, 98.3604) centre (121.524, 91.698) ccw projected
  arc A390 (118.0789, 98.4516) -> (118.3421, 98.9946) centre (117.8517, 98.897) ccw projected
  arc A391 (118.3396, 99.0073) -> (118.3421, 98.9946) centre (148.5, 105) ccw projected
  arc A392 (118.3396, 99.0073) -> (117.8886, 99.4083) centre (117.8492, 98.9099) ccw projected
  arc A393 (117.6937, 99.4263) -> (117.8886, 99.4083) centre (118.487, 106.9662) ccw projected
  arc A394 (116.9195, 99.5386) -> (117.6937, 99.4263) centre (118.7279, 109.2789) ccw projected
  arc A395 (115.9174, 99.7681) -> (116.9195, 99.5386) centre (119.1715, 111.6767) ccw projected
  arc A396 (115.8016, 100.5484) -> (115.9174, 99.7681) centre (148.5, 105) ccw projected
  arc A397 (116.6939, 101.0589) -> (115.8016, 100.5484) centre (122.3726, 90.0972) ccw projected
  arc A398 (117.4022, 101.3911) -> (116.6939, 101.0589) centre (121.252, 92.263) ccw projected
  arc A399 (117.5836, 101.4649) -> (117.4022, 101.3911) centre (120.3501, 94.4061) ccw projected
  arc A400 (117.5836, 101.4649) -> (117.8987, 101.9796) centre (117.4011, 101.9304) ccw projected
  arc A401 (117.8974, 101.9924) -> (117.8987, 101.9796) centre (148.5, 105) ccw projected
  arc A402 (117.8974, 101.9924) -> (117.488, 102.4357) centre (117.3998, 101.9435) ccw projected
  arc A403 (117.2957, 102.4727) -> (117.488, 102.4357) centre (118.8242, 109.8985) ccw projected
  arc A404 (116.5362, 102.6603) -> (117.2957, 102.4727) centre (119.2907, 112.1764) ccw projected
  arc A405 (115.5615, 102.9869) -> (116.5362, 102.6603) centre (119.9672, 114.5193) ccw projected
  arc A406 (115.5227, 103.7749) -> (115.5615, 102.9869) centre (148.5, 105) ccw projected
  arc A407 (116.4608, 104.1954) -> (115.5227, 103.7749) centre (121.0376, 92.7299) ccw projected
  arc A408 (117.1983, 104.4566) -> (116.4608, 104.1954) centre (120.1347, 94.9951) ccw projected
  arc A409 (117.3859, 104.5123) -> (117.1983, 104.4566) centre (119.4473, 97.2163) ccw projected
  arc A410 (117.3859, 104.5123) -> (117.75, 104.9935) centre (117.25, 104.9934) ccw projected
  arc A411 (117.75, 105.0065) -> (117.75, 104.9935) centre (148.5, 105) ccw projected
  arc A412 (117.75, 105.0065) -> (117.3859, 105.4877) centre (117.25, 105.0066) ccw projected
  arc A413 (117.1983, 105.5434) -> (117.3859, 105.4877) centre (119.4473, 112.7837) ccw projected
  arc A414 (116.4608, 105.8046) -> (117.1983, 105.5434) centre (120.1347, 115.0049) ccw projected
  arc A415 (115.5227, 106.2251) -> (116.4608, 105.8046) centre (121.0376, 117.2701) ccw projected
  arc A416 (115.5615, 107.0131) -> (115.5227, 106.2251) centre (148.5, 105) ccw projected
  arc A417 (116.5362, 107.3397) -> (115.5615, 107.0131) centre (119.9672, 95.4807) ccw projected
  arc A418 (117.2957, 107.5273) -> (116.5362, 107.3397) centre (119.2907, 97.8236) ccw projected
  arc A419 (117.488, 107.5643) -> (117.2957, 107.5273) centre (118.8242, 100.1015) ccw projected
  arc A420 (117.488, 107.5643) -> (117.8974, 108.0076) centre (117.3998, 108.0565) ccw projected
  arc A421 (117.8987, 108.0204) -> (117.8974, 108.0076) centre (148.5, 105) ccw projected
  arc A422 (117.8987, 108.0204) -> (117.5836, 108.5351) centre (117.4011, 108.0696) ccw projected
  arc A423 (117.4022, 108.6089) -> (117.5836, 108.5351) centre (120.3501, 115.5939) ccw projected
  arc A424 (116.6939, 108.9411) -> (117.4022, 108.6089) centre (121.252, 117.737) ccw projected
  arc A425 (115.8016, 109.4516) -> (116.6939, 108.9411) centre (122.3726, 119.9028) ccw projected
  arc A426 (115.9174, 110.2319) -> (115.8016, 109.4516) centre (148.5, 105) ccw projected
  arc A427 (116.9195, 110.4614) -> (115.9174, 110.2319) centre (119.1715, 98.3233) ccw projected
  arc A428 (117.6937, 110.5737) -> (116.9195, 110.4614) centre (118.7279, 100.7211) ccw projected
  arc A429 (117.8886, 110.5917) -> (117.6937, 110.5737) centre (118.487, 103.0338) ccw projected
  arc A430 (117.8886, 110.5917) -> (118.3396, 110.9927) centre (117.8492, 111.0901) ccw projected
  arc A431 (118.3421, 111.0054) -> (118.3396, 110.9927) centre (148.5, 105) ccw projected
  arc A432 (118.3421, 111.0054) -> (118.0789, 111.5484) centre (117.8517, 111.103) ccw projected
  arc A433 (117.9057, 111.6396) -> (118.0789, 111.5484) centre (121.524, 118.302) ccw projected
  arc A434 (117.2334, 112.0397) -> (117.9057, 111.6396) centre (122.6316, 120.3464) ccw projected
  arc A435 (116.3954, 112.6351) -> (117.2334, 112.0397) centre (123.9591, 122.392) ccw projected
  arc A436 (116.5871, 113.4004) -> (116.3954, 112.6351) centre (148.5, 105) ccw projected
  arc A437 (117.6068, 113.5305) -> (116.5871, 113.4004) centre (118.6583, 101.2301) ccw projected
  arc A438 (118.3884, 113.5664) -> (117.6068, 113.5305) centre (118.4519, 103.6599) ccw projected
  arc A439 (118.5841, 113.5652) -> (118.3884, 113.5664) centre (118.4388, 105.985) ccw projected
  arc A440 (118.5841, 113.5652) -> (119.0722, 113.9201) centre (118.5937, 114.0651) ccw projected
  arc A441 (119.076, 113.9324) -> (119.0722, 113.9201) centre (148.5, 105) ccw projected
  arc A442 (119.076, 113.9324) -> (118.8673, 114.4987) centre (118.5975, 114.0777) ccw projected
  arc A443 (118.7038, 114.6064) -> (118.8673, 114.4987) centre (122.9578, 120.8821) ccw projected
  arc A444 (118.074, 115.0704) -> (118.7038, 114.6064) centre (124.2604, 122.8081) ccw projected
  arc A445 (117.2984, 115.7452) -> (118.074, 115.0704) centre (125.782, 124.7137) ccw projected
  arc A446 (117.5642, 116.488) -> (117.2984, 115.7452) centre (148.5, 105) ccw projected
  arc A447 (118.5917, 116.5175) -> (117.5642, 116.488) centre (118.4325, 104.1733) ccw projected
  arc A448 (119.373, 116.4766) -> (118.5917, 116.5175) centre (118.4652, 106.6116) ccw projected
  arc A449 (119.5677, 116.4562) -> (119.373, 116.4766) centre (118.6801, 108.9268) ccw projected
  arc A450 (119.5677, 116.4562) -> (120.0882, 116.7616) centre (119.6263, 116.9528) ccw projected
  arc A451 (120.0932, 116.7735) -> (120.0882, 116.7616) centre (148.5, 105) ccw projected
  arc A452 (120.0932, 116.7735) -> (119.941, 117.3574) centre (119.6313, 116.9649) ccw projected
  arc A453 (119.7889, 117.4807) -> (119.941, 117.3574) centre (124.6375, 123.3092) ccw projected
  arc A454 (119.2076, 118.0042) -> (119.7889, 117.4807) centre (126.1226, 125.0982) ccw projected
  arc A455 (118.5018, 118.7517) -> (119.2076, 118.0042) centre (127.8237, 126.8455) ccw projected
  arc A456 (118.8391, 119.4649) -> (118.5018, 118.7517) centre (148.5, 105) ccw projected
  arc A457 (119.8647, 119.3936) -> (118.8391, 119.4649) centre (118.4963, 107.1244) ccw projected
  arc A458 (120.6382, 119.2763) -> (119.8647, 119.3936) centre (118.7678, 109.5478) ccw projected
  arc A459 (120.8299, 119.2369) -> (120.6382, 119.2763) centre (119.2086, 111.8308) ccw projected
  arc A460 (120.8299, 119.2369) -> (121.3779, 119.4898) centre (120.9369, 119.7254) ccw projected
  arc A461 (121.384, 119.5011) -> (121.3779, 119.4898) centre (148.5, 105) ccw projected
  arc A462 (121.384, 119.5011) -> (121.2898, 120.0972) centre (120.9431, 119.7369) ccw projected
  arc A463 (121.1505, 120.2348) -> (121.2898, 120.0972) centre (126.547, 125.56) ccw projected
  arc A464 (120.6232, 120.8128) -> (121.1505, 120.2348) centre (128.2004, 127.1948) ccw projected
  arc A465 (119.9942, 121.6258) -> (120.6232, 120.8128) centre (130.0645, 128.767) ccw projected
  arc A466 (120.3998, 122.3025) -> (119.9942, 121.6258) centre (148.5, 105) ccw projected
  arc A467 (121.4134, 122.131) -> (120.3998, 122.3025) centre (118.849, 110.055) ccw projected
  arc A468 (122.1717, 121.9385) -> (121.4134, 122.131) centre (119.3567, 112.4401) ccw projected
  arc A469 (122.3586, 121.8805) -> (122.1717, 121.9385) centre (120.0191, 114.6689) ccw projected
  arc A470 (122.3586, 121.8805) -> (122.9287, 122.0784) centre (122.5129, 122.3561) ccw projected
  arc A471 (122.9359, 122.0891) -> (122.9287, 122.0784) centre (148.5, 105) ccw projected
  arc A472 (122.9359, 122.0891) -> (122.9006, 122.6916) centre (122.5202, 122.367) ccw projected
  arc A473 (122.7754, 122.8421) -> (122.9006, 122.6916) centre (128.6679, 127.6127) ccw projected
  arc A474 (122.3074, 123.469) -> (122.7754, 122.8421) centre (130.4736, 129.0776) ccw projected
  arc A475 (121.7611, 124.3398) -> (122.3074, 123.469) centre (132.4828, 130.4595) ccw projected
  arc A476 (122.231, 124.9735) -> (121.7611, 124.3398) centre (148.5, 105) ccw projected
  arc A477 (123.2229, 124.7035) -> (122.231, 124.9735) centre (119.4872, 112.937) ccw projected
  arc A478 (123.9587, 124.4376) -> (123.2229, 124.7035) centre (120.2263, 115.2608) ccw projected
  arc A479 (124.1391, 124.3615) -> (123.9587, 124.4376) centre (121.104, 117.414) ccw projected
  arc A480 (124.1391, 124.3615) -> (124.7258, 124.5026) centre (124.3393, 124.8197) ccw projected
  arc A481 (124.734, 124.5126) -> (124.7258, 124.5026) centre (148.5, 105) ccw projected
  arc A482 (124.734, 124.5126) -> (124.7579, 125.1156) centre (124.3476, 124.8299) ccw projected
  arc A483 (124.6481, 125.2777) -> (124.7579, 125.1156) centre (130.9799, 129.4477) ccw projected
  arc A484 (124.2438, 125.9474) -> (124.6481, 125.2777) centre (132.9204, 130.7286) ccw projected
  arc A485 (123.7855, 126.8676) -> (124.2438, 125.9474) centre (135.0554, 131.9069) ccw projected
  arc A486 (124.3153, 127.4521) -> (123.7855, 126.8676) centre (148.5, 105) ccw projected
  arc A487 (125.2759, 127.0862) -> (124.3153, 127.4521) centre (120.4049, 115.7425) ccw projected
  arc A488 (125.9821, 126.7495) -> (125.2759, 127.0862) centre (121.3682, 117.9827) ccw projected
  arc A489 (126.1542, 126.6561) -> (125.9821, 126.7495) centre (122.4527, 120.0395) ccw projected
  arc A490 (126.1542, 126.6561) -> (126.7519, 126.739) centre (126.3983, 127.0924) ccw projected
  arc A491 (126.761, 126.7481) -> (126.7519, 126.739) centre (148.5, 105) ccw projected
  arc A492 (126.761, 126.7481) -> (126.8439, 127.3458) centre (126.4076, 127.1017) ccw projected
  arc A493 (126.7505, 127.5179) -> (126.8439, 127.3458) centre (133.4605, 131.0473) ccw projected
  arc A494 (126.4138, 128.2241) -> (126.7505, 127.5179) centre (135.5173, 132.1318) ccw projected
  arc A495 (126.0479, 129.1847) -> (126.4138, 128.2241) centre (137.7575, 133.0951) ccw projected
  arc A496 (126.6324, 129.7145) -> (126.0479, 129.1847) centre (148.5, 105) ccw projected
  arc A497 (127.5526, 129.2562) -> (126.6324, 129.7145) centre (121.5931, 118.4446) ccw projected
  arc A498 (128.2223, 128.8519) -> (127.5526, 129.2562) centre (122.7714, 120.5796) ccw projected
  arc A499 (128.3844, 128.7421) -> (128.2223, 128.8519) centre (124.0523, 122.5201) ccw projected
  arc A500 (128.3844, 128.7421) -> (128.9874, 128.766) centre (128.6701, 129.1524) ccw projected
  arc A501 (128.9974, 128.7742) -> (128.9874, 128.766) centre (148.5, 105) ccw projected
  arc A502 (128.9974, 128.7742) -> (129.1385, 129.3609) centre (128.6803, 129.1607) ccw projected
  arc A503 (129.0624, 129.5413) -> (129.1385, 129.3609) centre (136.086, 132.396) ccw projected
  arc A504 (128.7965, 130.2771) -> (129.0624, 129.5413) centre (138.2392, 133.2737) ccw projected
  arc A505 (128.5265, 131.269) -> (128.7965, 130.2771) centre (140.563, 134.0128) ccw projected
  arc A506 (129.1602, 131.7389) -> (128.5265, 131.269) centre (148.5, 105) ccw projected
  arc A507 (130.031, 131.1926) -> (129.1602, 131.7389) centre (123.0405, 121.0172) ccw projected
  arc A508 (130.6579, 130.7246) -> (130.031, 131.1926) centre (124.4224, 123.0264) ccw projected
  arc A509 (130.8084, 130.5994) -> (130.6579, 130.7246) centre (125.8873, 124.8321) ccw projected
  arc A510 (130.8084, 130.5994) -> (131.4109, 130.5641) centre (131.133, 130.9798) ccw projected
  arc A511 (131.4216, 130.5713) -> (131.4109, 130.5641) centre (148.5, 105) ccw projected
  arc A512 (131.4216, 130.5713) -> (131.6195, 131.1414) centre (131.1439, 130.9871) ccw projected
  arc A513 (131.5615, 131.3283) -> (131.6195, 131.1414) centre (138.8311, 133.4809) ccw projected
  arc A514 (131.369, 132.0866) -> (131.5615, 131.3283) centre (141.0599, 134.1433) ccw projected
  arc A515 (131.1975, 133.1002) -> (131.369, 132.0866) centre (143.445, 134.651) ccw projected
  arc A516 (131.8742, 133.5058) -> (131.1975, 133.1002) centre (148.5, 105) ccw projected
  arc A517 (132.6872, 132.8768) -> (131.8742, 133.5058) centre (124.733, 123.4355) ccw projected
  arc A518 (133.2652, 132.3495) -> (132.6872, 132.8768) centre (126.3052, 125.2996) ccw projected
  arc A519 (133.4028, 132.2102) -> (133.2652, 132.3495) centre (127.94, 126.953) ccw projected
  arc A520 (133.4028, 132.2102) -> (133.9989, 132.116) centre (133.7631, 132.5569) ccw projected
  arc A521 (134.0102, 132.1221) -> (133.9989, 132.116) centre (148.5, 105) ccw projected
  arc A522 (134.0102, 132.1221) -> (134.2631, 132.6701) centre (133.7746, 132.5631) ccw projected
  arc A523 (134.2237, 132.8618) -> (134.2631, 132.6701) centre (141.6692, 134.2914) ccw projected
  arc A524 (134.1064, 133.6353) -> (134.2237, 132.8618) centre (143.9522, 134.7322) ccw projected
  arc A525 (134.0351, 134.6609) -> (134.1064, 133.6353) centre (146.3756, 135.0037) ccw projected
  arc A526 (134.7483, 134.9982) -> (134.0351, 134.6609) centre (148.5, 105) ccw projected
  arc A527 (135.4958, 134.2924) -> (134.7483, 134.9982) centre (126.6545, 125.6763) ccw projected
  arc A528 (136.0193, 133.7111) -> (135.4958, 134.2924) centre (128.4018, 127.3774) ccw projected
  arc A529 (136.1426, 133.559) -> (136.0193, 133.7111) centre (130.1908, 128.8625) ccw projected
  arc A530 (136.1426, 133.559) -> (136.7265, 133.4068) centre (136.5351, 133.8687) ccw projected
  arc A531 (136.7384, 133.4118) -> (136.7265, 133.4068) centre (148.5, 105) ccw projected
  arc A532 (136.7384, 133.4118) -> (137.0438, 133.9323) centre (136.5472, 133.8737) ccw projected
  arc A533 (137.0234, 134.127) -> (137.0438, 133.9323) centre (144.5732, 134.8199) ccw projected
  arc A534 (136.9825, 134.9083) -> (137.0234, 134.127) centre (146.8884, 135.0348) ccw projected
  arc A535 (137.012, 135.9358) -> (136.9825, 134.9083) centre (149.3267, 135.0675) ccw projected
  arc A536 (137.7548, 136.2016) -> (137.012, 135.9358) centre (148.5, 105) ccw projected
  arc A537 (138.4296, 135.426) -> (137.7548, 136.2016) centre (128.7863, 127.718) ccw projected
  arc A538 (138.8936, 134.7962) -> (138.4296, 135.426) centre (130.6919, 129.2396) ccw projected
  arc A539 (139.0013, 134.6327) -> (138.8936, 134.7962) centre (132.6179, 130.5422) ccw projected
  arc A540 (139.0013, 134.6327) -> (139.5676, 134.424) centre (139.4223, 134.9025) ccw projected
  arc A541 (139.5799, 134.4278) -> (139.5676, 134.424) centre (148.5, 105) ccw projected
  arc A542 (139.5799, 134.4278) -> (139.9348, 134.9159) centre (139.4349, 134.9063) ccw projected
  arc A543 (139.9336, 135.1116) -> (139.9348, 134.9159) centre (147.515, 135.0612) ccw projected
  arc A544 (139.9695, 135.8932) -> (139.9336, 135.1116) centre (149.8401, 135.0481) ccw projected